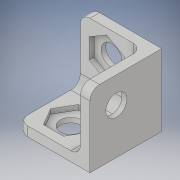
# Autodesk Inventor part: 23 bevestigings hoekjes 3 kanten
Saved by Autodesk Inventor 2019 (Build 230136000, 136)
## iProperties
Created: 2021-04-28
Part Number: 23 bevestigings hoekjes 3 kanten
Material: Generic
Document SubType Name: Modeling
Designer: Stefan
Density: 1 g/cm^3
Appearance: Default
Author: Stefan
Autodesk Inventor part; units mm, degrees
ref_plane "YZ Plane" through (0, 0, 0) normal (1, 0, 0) x (0, 1, 0)
ref_plane "XZ Plane" through (0, 0, 0) normal (0, 1, 0) x (-1, 0, 0)
ref_plane "XY Plane" through (0, 0, 0) normal (0, 0, 1) x (1, 0, 0)
sketch "Sketch1" plane through (0, 0, 0) normal (0, 0, 1) x (1, 0, 0)
  line L0 (-7.5, -7.5) -> (7.5, -7.5)
  line L1 (7.5, -7.5) -> (7.5, 7.5)
  line L2 (7.5, 7.5) -> (-7.5, 7.5)
  line L3 (-7.5, 7.5) -> (-7.5, -7.5)
  line L4 (-7.5, -7.5) -> (7.5, 7.5) construction
  line L5 (7.5, -7.5) -> (-7.5, 7.5) construction
  point P0 (0, 0)
  dimension "d0" = 15
  dimension "d1" = 15
  constraints: 12 end point, 2 midpoint, 2 parallel, 1 horizontal, 1 perpendicular
  measures "d0" distance of L2.end L1.end
  measures "d1" distance of L1.end L0.end
extrude "Extrusion1" add sketch "Sketch1" along normal blind 15
sketch "Sketch2" plane through (0, 0, 15) normal (0, 0, 1) x (1, 0, 0)
  line L0 (-7.5, 7.5) -> (-7.5, -7.5) projected
  line L1 (-7.5, 7.5) -> (5.5, 7.5)
  line L2 (5.5, 7.5) -> (5.5, -5.5)
  line L3 (5.5, -5.5) -> (-7.5, -5.5)
  line L4 (-7.5, -5.5) -> (-7.5, 7.5)
  line L5 (7.5, -7.5) -> (7.5, 7.5) projected
  line L6 (-7.5, -7.5) -> (7.5, -7.5) projected
  point P0 (0, 0)
  dimension "d4" = 2
  dimension "d5" = 2
  constraints: 8 end point, 2 parallel, 1 horizontal, 1 perpendicular
  measures "d4" distance between parallel lines of L5 L2
  measures "d5" distance between parallel lines of L6 L3
extrude "Extrusion2" cut sketch "Sketch2" against normal blind 13
sketch "Sketch6" plane through (5.5, -5.5, 15) normal (-1, 0, 0) x (0, 0, 1)
  line L0 (-5.5, 11.7147) -> (-1.85, 9.6073)
  line L1 (-1.85, 9.6073) -> (-1.85, 5.3927)
  line L2 (-1.85, 5.3927) -> (-5.5, 3.2853)
  line L3 (-5.5, 3.2853) -> (-9.15, 5.3927)
  line L4 (-9.15, 5.3927) -> (-9.15, 9.6073)
  line L5 (-9.15, 9.6073) -> (-5.5, 11.7147)
  line L6 (0, 0) -> (-13, 0) projected
  line L7 (-13, 0) -> (-13, 13) projected
  line L8 (0, 13) -> (0, 0) projected
  point P0 (-15, 5.5)
  point P1 (-5.5, 7.5)
  dimension "d41" = 7.5
  dimension "d42" = 7.5
  dimension "d43" = 7.3
  dimension "d44" = 0
  constraints: 12 end point, 13 other
  measures "d41" distance from line of L6 point (-5.5, 7.5)
  measures "d42" distance from line of L7 point (-5.5, 7.5)
  measures "d43" distance between parallel lines of L1 L4
  measures "d44" angle of L8 L1
extrude "Extrusion3" cut sketch "Sketch6" against normal blind 1
sketch "Sketch7" plane through (6.5, -5.5, 15) normal (-1, 0, 0) x (0, 0, 1)
  circle A0 centre (-5.5, 7.5) radius 2.2
  line L0 (0, 0) -> (-13, 0) projected
  line L1 (-13, 0) -> (-13, 13) projected
  point P0 (-15, 5.5)
  dimension "d47" = 4.4
  dimension "d48" = 7.5
  dimension "d49" = 7.5
  constraints: 1 centre point
  measures "d47" diameter of A0
  measures "d48" distance from line of L0 A0.centre
  measures "d49" distance from line of L1 A0.centre
extrude "Extrusion4" cut sketch "Sketch7" against normal blind 1
sketch "Sketch8" plane through (-7.5, -5.5, 15) normal (0, 1, 0) x (1, 0, 0)
  line L0 (3.3927, 1.85) -> (1.2853, 5.5)
  line L1 (1.2853, 5.5) -> (3.3927, 9.15)
  line L2 (3.3927, 9.15) -> (7.6073, 9.15)
  line L3 (7.6073, 9.15) -> (9.7147, 5.5)
  line L4 (9.7147, 5.5) -> (7.6073, 1.85)
  line L5 (7.6073, 1.85) -> (3.3927, 1.85)
  line L6 (0, 13) -> (13, 13) projected
  line L7 (13, 13) -> (13, 0) projected
  line L8 (13, 0) -> (0, 0) projected
  point P0 (7.5, 15)
  point P1 (5.5, 5.5)
  dimension "d52" = 7.3
  dimension "d53" = 7.5
  dimension "d54" = 7.5
  dimension "d55" = 0
  constraints: 12 end point, 13 other
  measures "d52" distance between parallel lines of L5 L2
  measures "d53" distance from line of L6 point (5.5, 5.5)
  measures "d54" distance from line of L7 point (5.5, 5.5)
  measures "d55" angle of L8 L5
extrude "Extrusion5" cut sketch "Sketch8" against normal blind 1
sketch "Sketch9" plane through (-7.5, -6.5, 15) normal (0, 1, 0) x (1, 0, 0)
  circle A0 centre (5.5, 5.5) radius 2.2
  line L0 (0, 13) -> (13, 13) projected
  line L1 (0, 0) -> (0, 13) projected
  point P0 (7.5, 15)
  dimension "d58" = 4.4
  dimension "d59" = 7.5
  dimension "d60" = 5.5
  constraints: 1 centre point
  measures "d58" diameter of A0
  measures "d59" distance from line of L0 A0.centre
  measures "d60" distance from line of L1 A0.centre
extrude "Extrusion6" cut sketch "Sketch9" against normal blind 1
sketch "Sketch10" plane through (0, 0, 2) normal (0, 0, 1) x (1, 0, 0)
  line L0 (1.65, -0.1073) -> (-2, -2.2147)
  line L1 (-2, -2.2147) -> (-5.65, -0.1073)
  line L2 (-5.65, -0.1073) -> (-5.65, 4.1073)
  line L3 (-5.65, 4.1073) -> (-2, 6.2147)
  line L4 (-2, 6.2147) -> (1.65, 4.1073)
  line L5 (1.65, 4.1073) -> (1.65, -0.1073)
  line L6 (5.5, -5.5) -> (-7.5, -5.5) projected
  line L7 (5.5, 7.5) -> (5.5, -5.5) projected
  line L8 (-7.5, -5.5) -> (-7.5, 7.5) projected
  point P0 (0, 0)
  point P1 (-2, 2)
  dimension "d63" = 7.5
  dimension "d64" = 7.5
  dimension "d65" = 7.3
  dimension "d66" = 0
  constraints: 12 end point, 13 other
  measures "d63" distance from line of L6 point (-2, 2)
  measures "d64" distance from line of L7 point (-2, 2)
  measures "d65" distance between parallel lines of L5 L2
  measures "d66" angle of L8 L2
extrude "Extrusion7" cut sketch "Sketch10" against normal blind 1
sketch "Sketch11" plane through (0, 0, 1) normal (0, 0, 1) x (1, 0, 0)
  circle A0 centre (-2, 2) radius 2.2
  line L0 (5.5, 7.5) -> (5.5, -5.5) projected
  line L1 (5.5, -5.5) -> (-7.5, -5.5) projected
  point P0 (0, 0)
  dimension "d69" = 4.4
  dimension "d70" = 7.5
  dimension "d71" = 7.5
  constraints: 1 centre point
  measures "d69" diameter of A0
  measures "d70" distance from line of L0 A0.centre
  measures "d71" distance from line of L1 A0.centre
extrude "Extrusion8" cut sketch "Sketch11" against normal blind 1
fillet "Fillet2" radius 2 3 edges at (-1, -5.5, 2) (5.5, -5.5, 8.5) (5.5, 1, 2)
fillet "Fillet3" radius 2 3 edges at (-7.5, 7.5, 1) (6.5, 7.5, 15) (-7.5, -6.5, 15)
body "Solid1"
